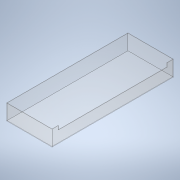
# Autodesk Inventor part: ElectricalBoard.ver2-1111-2020
Saved by Autodesk Inventor 2021 (Build 250183000, 183)
## iProperties
Created: 2020-01-21
Part Number: ElectricalBoard.ver2-1111-2020
Material: Generic
Document SubType Name: Modeling
Designer: JMHal
Density: 1 g/cm^3
Appearance: Polycarbonate - Clear
Author: JMHal
Autodesk Inventor part; units mm, degrees
ref_plane "YZ Plane" through (0, 0, 0) normal (1, 0, 0) x (0, 1, 0)
ref_plane "XZ Plane" through (0, 0, 0) normal (0, 1, 0) x (-1, 0, 0)
ref_plane "XY Plane" through (0, 0, 0) normal (0, 0, 1) x (1, 0, 0)
sketch "Sketch2" plane through (0, 0, 0) normal (0, 1, 0) x (-1, 0, 0)
  line L0 (0, 0) -> (914.4, 0)
  line L1 (914.4, 0) -> (914.4, -2438.4)
  line L2 (914.4, -2438.4) -> (0, -2438.4)
  line L3 (0, -2438.4) -> (0, 0)
  dimension "d22" = 2438.4
  dimension "d23" = 914.4
  constraints: 8 end point, 2 parallel, 1 horizontal, 1 perpendicular
  measures "d22" distance between parallel lines of L2 L0
  measures "d23" distance between parallel lines of L1 L3
extrude "Extrusion2" add sketch "Sketch2" along normal blind 6.35
sketch "Sketch3" plane through (0, 6.35, 0) normal (0, 1, 0) x (1, 0, 0)
  line L0 (-914.4, 2438.4) -> (-914.4, 0) projected
  line L1 (0, 2438.4) -> (-914.4, 2438.4) projected
  line L2 (-914.4, 0) -> (0, 0)
  line L3 (0, 0) -> (0, 2438.4)
  line L4 (0, 2438.4) -> (-914.4, 2438.4)
  line L5 (-914.4, 2438.4) -> (-914.4, 0)
  line L6 (-6.35, 6.35) -> (-908.05, 6.35)
  line L7 (-908.05, 6.35) -> (-908.05, 2432.05)
  line L8 (-908.05, 2432.05) -> (-6.35, 2432.05)
  line L9 (-6.35, 2432.05) -> (-6.35, 6.35)
  dimension "d24" = 6.35
  constraints: 16 end point, 4 parallel, 2 perpendicular, 1 horizontal, 3 other
  measures "d24" distance between parallel lines of L2 L6
extrude "Extrusion3" add sketch "Sketch3" along normal blind 304.8
sketch "Sketch4" plane through (0, 0, 0) normal (1, 0, 0) x (0, 0, -1)
  line L0 (0, 0) -> (0, 311.15) projected
  line L1 (2438.4, 0) -> (2438.4, 311.15) projected
  line L2 (0, 311.15) -> (2438.4, 311.15)
  line L3 (2438.4, 311.15) -> (2311.4, 311.15)
  line L4 (2432.05, 311.15) -> (6.35, 311.15) projected
  line L5 (0, 311.15) -> (127, 311.15)
  line L6 (127, 311.15) -> (127, 234.95)
  line L7 (127, 234.95) -> (2311.4, 234.95)
  line L8 (2311.4, 234.95) -> (2311.4, 311.15)
  dimension "d27" = 127
  dimension "d28" = 127
  dimension "d29" = 76.2
  constraints: 12 end point, 2 perpendicular, 2 point on line, 1 horizontal, 1 vertical
  measures "d27" distance of L1.end L3.end
  measures "d28" distance of L0.end L5.end
  measures "d29" distance of L5.end L6.end
extrude "Extrusion4" cut sketch "Sketch4" against normal blind 50.8
body "Solid2"
